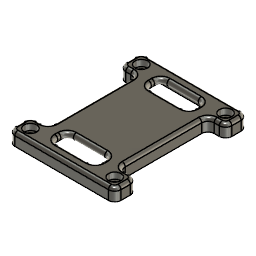
Battery Monitor Assembly (Autodesk Fusion 360 archive; units mm, degrees)
design "Lid"
part number: 2026-03-17-17-51-11-445
Autodesk Fusion 360 part; units mm, degrees
sketch "Bottom" plane through (0, 0, 0) normal (0, 0, 1) x (1, 0, 0)
  line L0 (17, 21.25) -> (-17, 21.25)
  line L1 (-17, 21.25) -> (-17, -21.25)
  line L2 (-17, -21.25) -> (17, -21.25)
  line L3 (17, -21.25) -> (17, 21.25)
  line L4 (17, 21.25) -> (-17, -21.25) construction
  line L5 (-17, 21.25) -> (17, -21.25) construction
  line L6 (17, 21.25) -> (10, 21.25)
  line L7 (10, 21.25) -> (10, 14.25)
  line L8 (10, 14.25) -> (17, 14.25)
  line L9 (17, 14.25) -> (17, 21.25)
  circle A0 centre (13.5, 17.75) radius 1.15
  circle A1 centre (13.5, 17.75) radius 2
  circle A2 centre (-13.5, 17.75) radius 2
  circle A3 centre (-13.5, 17.75) radius 1.15
  line L10 (-17, 14.25) -> (-10, 14.25)
  line L11 (-17, 21.25) -> (-17, 14.25)
  line L12 (-10, 21.25) -> (-17, 21.25)
  line L13 (-10, 14.25) -> (-10, 21.25)
  circle A4 centre (13.5, -17.75) radius 2
  circle A5 centre (13.5, -17.75) radius 1.15
  line L14 (10, -21.25) -> (17, -21.25)
  line L15 (10, -14.25) -> (10, -21.25)
  line L16 (17, -14.25) -> (10, -14.25)
  line L17 (17, -21.25) -> (17, -14.25)
  circle A6 centre (-13.5, -17.75) radius 2
  circle A7 centre (-13.5, -17.75) radius 1.15
  line L18 (-17, -21.25) -> (-10, -21.25)
  line L19 (-17, -14.25) -> (-17, -21.25)
  line L20 (-10, -14.25) -> (-17, -14.25)
  line L21 (-10, -21.25) -> (-10, -14.25)
  line L22 (17, -14.25) -> (11.35, -14.25)
  line L23 (11.35, -14.25) -> (11.35, 14.25)
  line L24 (11.35, 14.25) -> (17, 14.25)
  line L25 (17, 14.25) -> (17, -14.25)
  line L26 (-17, -14.25) -> (-11.35, -14.25)
  line L27 (-11.35, -14.25) -> (-11.35, 14.25)
  line L28 (-11.35, 14.25) -> (-17, 14.25)
  line L29 (-17, 14.25) -> (-17, -14.25)
  line L30 (9.5, 19.5) -> (-9.5, 19.5)
  line L31 (-9.5, 19.5) -> (-9.5, -19.5)
  line L32 (-9.5, -19.5) -> (9.5, -19.5)
  line L33 (9.5, -19.5) -> (9.5, 19.5)
  line L34 (9.5, 19.5) -> (-9.5, -19.5) construction
  line L35 (-9.5, 19.5) -> (9.5, -19.5) construction
  dimension "d37" = 34
  dimension "d38" = 42.5
  dimension "d39" = 7
  dimension "d40" = 7
  dimension "d41" = 2.3
  dimension "d42" = 4
  dimension "d45" = -27
  dimension "d46" = -35.5
  dimension "d47" = 5.65
  dimension "d48" = 5.65
  dimension "d53" = 19
  dimension "d54" = 39
  constraint horizontal L0
  constraint perpendicular L0 L1
  constraint parallel L0 L2
  constraint parallel L1 L3
  constraint coincident L4 origin
  constraint coincident L5 origin
  constraint horizontal L6
  constraint vertical L7
  constraint horizontal L8
  constraint vertical L9
  constraint concentric A0 A1
  constraint horizontal L22
  constraint vertical L23
  constraint horizontal L24
  constraint vertical L25
  constraint horizontal L26
  constraint vertical L27
  constraint horizontal L28
  constraint vertical L29
  constraint horizontal L30
  constraint perpendicular L30 L31
  constraint parallel L30 L32
  constraint parallel L31 L33
  constraint coincident L34 origin
  constraint coincident L35 origin
  measures "d37" distance of L1.end L2.end
  measures "d38" distance of L0.end L1.end
  measures "d39" distance of L0.start L6.end
  measures "d40" distance of L0.start L8.end
  measures "d41" diameter of A0
  measures "d42" diameter of A1
  measures "d47" distance of L16.start L22.end
  measures "d48" distance of L19.start L26.end
  measures "d53" distance of L31.end L32.end
  measures "d54" distance of L30.end L31.end
extrude "Extrude5" add sketch "Bottom" along normal blind 4 contours L0 L3 L6 L7 L8 L9 L24 | L0 L2 L7 L8 L10 L13 L15 L16 L20 L21 L23 L27 | L0 L1 L10 L11 L12 L13 L28 | L2 L3 L14 L15 L16 L17 L22 | L1 L2 L18 L19 L20 L21 L26 | L30 L31 L32 L33
extrude "Extrude6" add sketch "Bottom" along normal blind 2 contours A1 | A2 | A4 | A6
extrude "Extrude7" cut sketch "Bottom" along normal blind 2 contours L30 L31 L32 L33
fillet "Fillet1" radius 2 12 edges at (11.35, 14.25, 2) (17, 14.25, 2) (17, 21.25, 2) (-17, 21.25, 2) (-17, 14.25, 2) (-11.35, 14.25, 2) (-11.35, -14.25, 2) (-17, -14.25, 2) (-17, -21.25, 2) (17, -21.25, 2) (17, -14.25, 2) (11.35, -14.25, 2)
sketch "Inside" plane through (0, 0, 2) normal (0, 0, -1) x (1, 0, 0)
  line L0 (9.5, -19.5) -> (9.5, 19.5)
  line L1 (9.5, 19.5) -> (-9.5, 19.5)
  line L2 (-9.5, 19.5) -> (-9.5, -19.5)
  line L3 (-9.5, -19.5) -> (9.5, -19.5)
  line L4 (-7, -12.5) -> (7, -12.5)
  line L5 (7, -12.5) -> (7, -17.5)
  line L6 (7, -17.5) -> (-7, -17.5)
  line L7 (-7, -17.5) -> (-7, -12.5)
  line L8 (-7, -12.5) -> (7, -17.5) construction
  line L9 (7, -12.5) -> (-7, -17.5) construction
  line L10 (-7, 17.5) -> (7, 17.5)
  line L11 (7, 17.5) -> (7, 12.5)
  line L12 (7, 12.5) -> (-7, 12.5)
  line L13 (-7, 12.5) -> (-7, 17.5)
  line L14 (-7, 17.5) -> (7, 12.5) construction
  line L15 (7, 17.5) -> (-7, 12.5) construction
  point P0 (0, -15)
  point P1 (0, 15)
  dimension "d71" = 14
  dimension "d72" = 5
  dimension "d73" = 14
  dimension "d74" = 5
  constraint horizontal L4
  constraint perpendicular L4 L5
  constraint parallel L4 L6
  constraint parallel L5 L7
  constraint coincident L8 P0
  constraint coincident L9 P0
  constraint horizontal L10
  constraint perpendicular L10 L11
  constraint parallel L10 L12
  constraint parallel L11 L13
  constraint coincident L14 P1
  constraint coincident L15 P1
  measures "d71" distance of L5.end L6.end
  measures "d72" distance of L4.end L5.end
  measures "d73" distance of L11.end L12.end
  measures "d74" distance of L10.end L11.end
extrude "Extrude10" cut sketch "Inside" against normal blind 2 contours L4 L5 L6 L7 | L10 L11 L12 L13
fillet "Fillet5" radius 2 8 edges at (-7, -17.5, 3) (-7, 12.5, 3) (-7, 17.5, 3) (7, 17.5, 3) (7, 12.5, 3) (7, -12.5, 3) (7, -17.5, 3) (-7, -12.5, 3)
fillet "Fillet6" radius 1 32 edges at (0, 12.5, 4) (6.4142, 13.0858, 4) (7, 15, 4) (6.4142, 16.9142, 4) (0, 17.5, 4) (-6.4142, 16.9142, 4) (-7, 15, 4) (-6.4142, 13.0858, 4) (-7, 15, 2) (-6.4142, 16.9142, 2) (0, 17.5, 2) (6.4142, 16.9142, 2) (7, 15, 2) (6.4142, 13.0858, 2) (0, 12.5, 2) (-6.4142, 13.0858, 2) (-6.4142, -13.0858, 2) (-7, -15, 2) (-6.4142, -16.9142, 2) (0, -17.5, 2) (6.4142, -16.9142, 2) (7, -15, 2) (6.4142, -13.0858, 2) (0, -12.5, 2) (6.4142, -13.0858, 4) (7, -15, 4) (6.4142, -16.9142, 4) (0, -17.5, 4) (-6.4142, -16.9142, 4) (-7, -15, 4) (-6.4142, -13.0858, 4) (0, -12.5, 4)
fillet "Fillet7" radius 1 24 edges at (-14.175, 14.25, 4) (-16.4142, 14.8358, 4) (-17, 17.75, 4) (-16.4142, 20.6642, 4) (0, 21.25, 4) (16.4142, 20.6642, 4) (17, 17.75, 4) (16.4142, 14.8358, 4) (14.175, 14.25, 4) (11.9358, 13.6642, 4) (11.35, 0, 4) (11.9358, -13.6642, 4) (14.175, -14.25, 4) (16.4142, -14.8358, 4) (17, -17.75, 4) (16.4142, -20.6642, 4) (0, -21.25, 4) (-16.4142, -20.6642, 4) (-17, -17.75, 4) (-16.4142, -14.8358, 4) (-14.175, -14.25, 4) (-11.9358, -13.6642, 4) (-11.35, 0, 4) (-11.9358, 13.6642, 4)

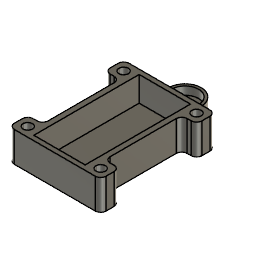
design "Mount"
part number: 2026-03-17-16-26-03-038
Autodesk Fusion 360 part; units mm, degrees
sketch "Bottom" plane through (0, 0, 0) normal (0, 0, 1) x (1, 0, 0)
  line L0 (9.5, 19.5) -> (-9.5, 19.5)
  line L1 (-9.5, 19.5) -> (-9.5, -19.5)
  line L2 (-9.5, -19.5) -> (9.5, -19.5)
  line L3 (9.5, -19.5) -> (9.5, 19.5)
  line L4 (9.5, 19.5) -> (-9.5, -19.5) construction
  line L5 (-9.5, 19.5) -> (9.5, -19.5) construction
  circle A0 centre (0, 27) radius 5
  circle A1 centre (0, 27) radius 2.75
  circle A2 centre (0, 27) radius 6
  spline S0 degree 5 poles (6, 27) (5.9999, 26.8077) (6.0067, 26.4298) (6.0375, 25.8828) (6.1205, 25.1941) (6.2992, 24.4054) (6.5597, 23.6957) (6.9094, 23.0721) (7.3531, 22.5393) (7.8885, 22.095) (8.5092, 21.7332) (9.0688, 21.5044) (9.5217, 21.365) (9.8381, 21.286) (10, 21.25) knots 0 0 0 0 0 0 0.1 0.2 0.3 0.4 0.5 0.6 0.7 0.8 0.9 1 1 1 1 1 1
  spline S1 degree 5 poles (-6, 27) (-5.9999, 26.8077) (-6.0067, 26.4298) (-6.0375, 25.8828) (-6.1205, 25.1941) (-6.2992, 24.4054) (-6.5597, 23.6957) (-6.9094, 23.0721) (-7.3531, 22.5393) (-7.8885, 22.095) (-8.5092, 21.7332) (-9.0688, 21.5044) (-9.5217, 21.365) (-9.8381, 21.286) (-10, 21.25) knots 0 0 0 0 0 0 0.1 0.2 0.3 0.4 0.5 0.6 0.7 0.8 0.9 1 1 1 1 1 1
  line L6 (17, 21.25) -> (-17, 21.25)
  line L7 (-17, 21.25) -> (-17, -21.25)
  line L8 (-17, -21.25) -> (17, -21.25)
  line L9 (17, -21.25) -> (17, 21.25)
  line L10 (17, 21.25) -> (-17, -21.25) construction
  line L11 (-17, 21.25) -> (17, -21.25) construction
  line L12 (17, 21.25) -> (13.5, 21.25)
  line L13 (13.5, 21.25) -> (13.5, 17.75)
  line L14 (13.5, 17.75) -> (17, 17.75)
  line L15 (17, 17.75) -> (17, 21.25)
  circle A3 centre (13.5, 17.75) radius 1.75
  circle A4 centre (-13.5, 17.75) radius 1.75
  circle A5 centre (13.5, -17.75) radius 1.75
  circle A6 centre (-13.5, -17.75) radius 1.75
  line L16 (17, -21.25) -> (10, -21.25)
  line L17 (10, -21.25) -> (10, -14.25)
  line L18 (10, -14.25) -> (17, -14.25)
  line L19 (17, -14.25) -> (17, -21.25)
  line L20 (17, -21.25) -> (10, -14.25) construction
  line L21 (10, -21.25) -> (17, -14.25) construction
  line L22 (17, 21.25) -> (10, 21.25)
  line L23 (10, 21.25) -> (10, 14.25)
  line L24 (10, 14.25) -> (17, 14.25)
  line L25 (17, 14.25) -> (17, 21.25)
  line L26 (17, 21.25) -> (10, 14.25) construction
  line L27 (10, 21.25) -> (17, 14.25) construction
  line L28 (10, 14.25) -> (17, 14.25)
  line L29 (17, 14.25) -> (17, -14.25)
  line L30 (17, -14.25) -> (10, -14.25)
  line L31 (-17, 14.25) -> (-10, 14.25)
  line L32 (-17, 21.25) -> (-17, 14.25)
  line L33 (-17, -14.25) -> (-17, 14.25)
  line L34 (-17, -21.25) -> (-17, -14.25)
  line L35 (-17, -14.25) -> (-10, -14.25)
  line L36 (-10, -21.25) -> (-10, 21.25)
  line L37 (9.5, -14.25) -> (11.5, -14.25)
  line L38 (11.5, -14.25) -> (11.5, 14.25)
  line L39 (11.5, 14.25) -> (9.5, 14.25)
  line L40 (9.5, 14.25) -> (9.5, -14.25)
  line L41 (-9.5, -14.25) -> (-11.5, -14.25)
  line L42 (-11.5, -14.25) -> (-11.5, 14.25)
  line L43 (-11.5, 14.25) -> (-9.5, 14.25)
  line L44 (-9.5, 14.25) -> (-9.5, -14.25)
  point P0 (7, 23)
  point P1 (-7, 23)
  point P2 (13.5, -17.75)
  point P3 (13.5, 17.75)
  dimension "d1" = 19
  dimension "d2" = 39
  dimension "d8" = 10
  dimension "d9" = 5.5
  dimension "d10" = 12
  dimension "d26" = 42.5
  dimension "d30" = 3.5
  dimension "d31" = 3.5
  dimension "d32" = 3.5
  dimension "d35" = -27
  dimension "d36" = -35.5
  dimension "d51" = 2
  dimension "d52" = 2
  constraint horizontal L0
  constraint perpendicular L0 L1
  constraint parallel L0 L2
  constraint parallel L1 L3
  constraint coincident L4 origin
  constraint coincident L5 origin
  constraint concentric A0 A1
  constraint concentric A1 A2
  constraint coincident A2 S0.start
  constraint coincident A2 S1.start
  constraint horizontal L6
  constraint perpendicular L6 L7
  constraint parallel L6 L8
  constraint parallel L7 L9
  constraint coincident L10 origin
  constraint coincident L11 origin
  constraint horizontal L12
  constraint vertical L13
  constraint horizontal L14
  constraint vertical L15
  constraint coincident P3 L13.end
  constraint horizontal L16
  constraint perpendicular L16 L17
  constraint parallel L16 L18
  constraint parallel L17 L19
  constraint coincident L20 P2
  constraint coincident L21 P2
  constraint coincident P2 A5.centre
  constraint horizontal L22
  constraint perpendicular L22 L23
  constraint parallel L22 L24
  constraint parallel L23 L25
  constraint coincident L26 P3
  constraint coincident L27 P3
  constraint horizontal L28
  constraint vertical L29
  constraint horizontal L30
  constraint horizontal L37
  constraint vertical L38
  constraint horizontal L39
  constraint vertical L40
  constraint coincident L3 L37.start
  constraint horizontal L41
  constraint vertical L42
  constraint horizontal L43
  constraint vertical L44
  constraint coincident L1 L41.start
  measures "d1" distance of L1.end L2.end
  measures "d2" distance of L0.end L1.end
  measures "d8" diameter of A0
  measures "d9" diameter of A1
  measures "d10" diameter of A2
  measures "d26" distance of L6.end L7.end
  measures "d30" distance of L6.start L12.end
  measures "d31" distance of L6.start L14.end
  measures "d32" diameter of A3
  measures "d51" distance of L37.start L37.end
  measures "d52" distance of L41.start L41.end
extrude "Extrude8" add sketch "Bottom" along normal blind 11.2 contours L0 L1 L3 A2 L6 L23 L36 L39 L43 | L3 L18 L24 L28 L30 L37 L38 L39 L40 | L1 L36 L41 L43 L44 | L1 L2 L3 L8 L17 L36 L37 L41 | L6 L9 L13 L14 A3 L22 L23 L24 L25 L28 L39 | L31 L35 L36 L41 L42 L43 | L6 L7 L31 L32 L36 L43 | L8 L9 L16 L17 L18 L19 L30 L37 | L7 L8 L34 L35 L36 L41 | L6 L9 L12 L13 L14 L15 A3 L22 L25 | A2 L6 picked at (0.2887, 21.1876) makes body 1
extrude "Extrude9" add sketch "Bottom" along normal blind 2 contours L0 L1 L2 L3 L40 L44 | A0 bodies 1 makes body 2 at (4.9938, 26.7508, 1.3333)
extrude "Extrude10" add sketch "Bottom" along normal blind 5 contours A2 S1 L6 | A2 L6 | A2 S0 L6 | L13 L14 A3 | L13 L14 A3 | A4 | A5 | A6 picked at (0.1246, 21.5047) bodies 1 2
fillet "Fillet3" radius 2 11 edges at (17, 14.25, 5.6) (11.5, 14.25, 5.6) (17, 21.25, 5.6) (-17, 21.25, 5.6) (-11.5, 14.25, 5.6) (-11.5, -14.25, 5.6) (-17, -14.25, 5.6) (-17, -21.25, 5.6) (17, -21.25, 5.6) (17, -14.25, 5.6) (11.5, -14.25, 5.6) on bodies 1
fillet "Fillet3" radius 2 1 edges at (-17, 14.25, 5.6) on bodies 1
